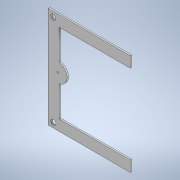
# Autodesk Inventor part: P8
Saved by Autodesk Inventor 2022 (Build 260153000, 153)
## iProperties
Created: 2022-11-16
Part Number: P8
Material: Genérico
Document SubType Name: Modeling
Designer: javie
Density: 1 g/cm^3
Appearance: Valor por defecto
Author: javie
Autodesk Inventor part; units mm, degrees
ref_plane "YZ Plane" through (0, 0, 0) normal (1, 0, 0) x (0, 1, 0)
ref_plane "XZ Plane" through (0, 0, 0) normal (0, 1, 0) x (-1, 0, 0)
ref_plane "XY Plane" through (0, 0, 0) normal (0, 0, 1) x (1, 0, 0)
sketch "Boceto1" plane through (0, 0, 0) normal (0, 0, 1) x (1, 0, 0)
  circle A0 centre (32.0216, 148.5297) radius 3.5
  line L0 (40.0216, 140.5297) -> (40.0216, 98.3749)
  line L1 (40.0216, 72.6844) -> (40.0216, 30.5297)
  line L2 (25.0216, 15.5297) -> (25.0216, 155.5297)
  line L3 (40.0216, 30.5297) -> (138.3848, 30.5297)
  line L4 (6.0787, 0.7542) -> (6.0787, 166.9226)
  line L5 (163.6392, 166.9226) -> (163.6392, 0.7542)
  line L6 (138.3848, 15.5297) -> (25.0216, 15.5297)
  line L7 (163.6392, 0.7542) -> (6.0787, 0.7542)
  arc A1 (40.0216, 72.6844) -> (40.0216, 98.3749) centre (38.0216, 85.5297) ccw
  line L8 (138.3848, 30.5297) -> (138.3848, 15.5297)
  line L9 (138.3848, 155.5297) -> (138.3848, 140.5297)
  line L10 (138.3848, 140.5297) -> (40.0216, 140.5297)
  line L11 (6.0787, 166.9226) -> (163.6392, 166.9226)
  line L12 (25.0216, 155.5297) -> (138.3848, 155.5297)
  circle A2 centre (32.0216, 22.5297) radius 3.5
  circle A3 centre (38.0216, 85.5297) radius 1
  point P0 (0, 0)
  point P1 (0, 0)
  point P2 (40.0216, 98.3749)
  dimension "d0" = 2
  constraints: 26 end point, 4 centre point, 2 point on circle, 1 coincident
  measures "d0" diameter of A3
extrude "Extrusión1" add sketch "Boceto1" along normal blind 2 contours L0 A1 L1 L3 L8 L6 L2 L12 L9 L10
